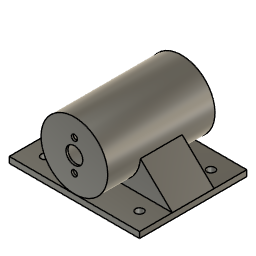
motor_support_v6 (Autodesk Fusion 360 design; units mm, degrees)
Autodesk Fusion 360 part; units mm, degrees
note: some values were not read from the file. Set by a fixed rule: which sketch regions a step uses.
sketch "Esboço1" plane through (0, 0, 0) normal (0, 1, 0) x (1, 0, 0)
  circle A0 centre (0, 7.75) radius 1.5
  circle A1 centre (0, -7.75) radius 1.5
  circle A2 centre (0, -0.0264) radius 4.25
  line L0 (0, 9.25) -> (0, 13.2236) construction
  line L1 (4.2485, 0.0836) -> (13.2495, 0.0836) construction
  line L2 (-4.2485, 0.0836) -> (-13.2495, 0.0836) construction
  line L3 (0.0108, -13.2764) -> (0.0108, -9.25) construction
  line L4 (0.0108, -6.25) -> (0.0108, -4.2764) construction
  line L5 (0.0108, 6.25) -> (0.0108, 4.2235) construction
  circle A3 centre (0, -0.0264) radius 14.25
  dimension "d3" = 3
  dimension "d5" = 3
  dimension "d73" = 8.4999
  dimension "d79" = 9.001
  dimension "d80" = 9.001
  dimension "d81" = 4.0265
  dimension "d82" = 1.9737
  dimension "d83" = 2.0265
  dimension "d84" = 3.9736
  dimension "d269" = 28.5
  constraint coincident A0 L0.start
  constraint vertical L0
  constraint coincident A2 L1.start
  constraint horizontal L1
  constraint coincident A2 L2.start
  constraint parallel L1 L2
  constraint coincident A1 L3.end
  constraint vertical L3
  constraint coincident A1 L4.start
  constraint coincident A2 L4.end
  constraint parallel L3 L4
  constraint coincident A0 L5.start
  constraint coincident A2 L5.end
  constraint parallel L4 L5
  measures "d3" diameter of A0
  measures "d5" diameter of A1
  measures "d73" diameter of A2
  measures "d79" distance of L1.start L1.end
  measures "d80" distance of L2.start L2.end
  measures "d81" distance of L3.start L3.end
  measures "d82" distance of L4.start L4.end
  measures "d83" distance of L5.start L5.end
  measures "d84" distance of L0.start L0.end
  measures "d269" diameter of A3
sketch "Esboço8" plane through (0, 0, 0) normal (0, 1, 0) x (1, 0, 0)
  circle A0 centre (0, 0) radius 16.8
  dimension "d87" = 33.6
  constraint coincident A0.centre origin
  measures "d87" diameter of A0
extrude "Extrusão14" add sketch "Esboço1" along normal blind 1
extrude "Extrusão15" add sketch "Esboço8" along normal blind 54 thin wall 3 inside
ref_plane "Plano de trabalho5" through (0, 27, 0) normal (0, 1, 0) x (1, 0, 0)
ref_plane "Plano de trabalho7" through (0, 33.6131, -16.8) normal (0, 0, -1) x (1, 0, 0)
sketch "Esboço14" plane through (0, 0, -16.8) normal (0, 0, -1) x (-1, 0, 0)
  line L0 (0, 0) -> (-15.8, 0)
  line L1 (0, 0) -> (15.8, 0)
  line L2 (0, 54) -> (-15.8, 54)
  line L3 (0, 54) -> (15.8, 54)
  line L4 (-15.8, 0) -> (-15.8, 54) construction
  line L5 (15.8, 0) -> (15.8, 54) construction
  line L6 (-15.8, 0) -> (-32.8, 0)
  line L7 (15.8, 0) -> (32.8, 0)
  line L8 (-15.8, 54) -> (-32.8, 54)
  line L9 (15.8, 54) -> (32.8, 54)
  line L10 (32.8, 0) -> (32.8, 54)
  line L11 (-32.8, 0) -> (-32.8, 54)
  line L12 (-32.8, 3) -> (-29.8, 3) construction
  line L13 (-29.8, 0) -> (-29.8, 3) construction
  circle A0 centre (-23.8, 9) radius 6 construction
  circle A1 centre (-23.8, 9) radius 2
  line L14 (-32.8, 27) -> (32.8, 27) construction
  line L15 (-32.8, 27) -> (32.8, 27) construction
  circle A2 centre (-23.8, 45) radius 6 construction
  circle A3 centre (-23.8, 45) radius 2
  line L16 (-29.8, 54) -> (-29.8, 51) construction
  line L17 (-32.8, 51) -> (-29.8, 51) construction
  line L18 (0, 0) -> (0, 54) construction
  circle A4 centre (23.8, 9) radius 2
  circle A5 centre (23.8, 9) radius 6 construction
  line L19 (32.8, 3) -> (29.8, 3) construction
  line L20 (29.8, 0) -> (29.8, 3) construction
  circle A6 centre (23.8, 45) radius 6 construction
  circle A7 centre (23.8, 45) radius 2
  line L21 (32.8, 51) -> (29.8, 51) construction
  line L22 (29.8, 54) -> (29.8, 51) construction
  dimension "d244" = 15.8
  dimension "d245" = 15.8
  dimension "d246" = 15.8
  dimension "d247" = 15.8
  dimension "d249" = 17
  dimension "d250" = 17
  dimension "d251" = 17
  dimension "d252" = 17
  dimension "d253" = 54
  dimension "d256" = 6
  dimension "d257" = 4
  dimension "d258" = 3
  dimension "d259" = 3
  constraint coincident L0.start L1.start
  constraint horizontal L0
  constraint parallel L0 L1
  constraint horizontal L2
  constraint parallel L2 L3
  constraint perpendicular L2 L4
  constraint perpendicular L4 L6
  constraint perpendicular L5 L7
  constraint perpendicular L4 L8
  constraint perpendicular L5 L9
  constraint coincident L11 L12.start
  constraint coincident L6 L13.start
  constraint perpendicular L12 L13
  constraint tangent L13 A0
  constraint concentric A0 A1
  constraint midpoint L11 L14.start
  constraint midpoint L10 L14.end
  constraint symmetric L12.start L14 L17.start
  constraint symmetric L12.end L14 L16.end
  constraint symmetric L13.start L14 L16.start
  constraint symmetric A0 L14 A2
  constraint symmetric A1 L14 A3
  constraint symmetric L15.start L14 L14.start
  constraint symmetric L15.end L14 L14.end
  constraint symmetric L12.start L18 L19.start
  constraint symmetric L12.end L18 L19.end
  constraint symmetric L13.start L18 L20.start
  constraint symmetric A0 L18 A5
  constraint symmetric A1 L18 A4
  constraint symmetric A2 L18 A6
  constraint symmetric A3 L18 A7
  constraint symmetric L16.start L18 L22.start
  constraint symmetric L16.end L18 L21.end
  constraint symmetric L17.start L18 L21.start
  measures "d244" distance of L0.start L0.end
  measures "d245" distance of L0.start L1.end
  measures "d246" distance of L2.start L2.end
  measures "d247" distance of L2.start L3.end
  measures "d249" distance of L0.end L6.end
  measures "d250" distance of L1.end L7.end
  measures "d251" distance of L2.end L8.end
  measures "d252" distance of L3.end L9.end
  measures "d253" distance of L6.end L8.end
  measures "d256" radius of A0
  measures "d257" diameter of A1
  measures "d258" distance of L12.end L13.start
  measures "d259" distance of L12.start L12.end
extrude "Extrusão19" add sketch "Esboço14" along normal blind 3
sketch "Esboço16" plane through (0, 27, 0) normal (0, 1, 0) x (1, 0, 0)
  line L0 (-15.7624, 0.308) -> (-15.7658, 1.0442) construction
  line L1 (-15.7658, 1.0442) -> (-15.5807, 1.9927) construction
  line L2 (-15.5807, 1.9927) -> (-15.3833, 3.1059) construction
  line L3 (-15.3833, 3.1059) -> (-14.9922, 4.8134) construction
  line L4 (-14.9922, 4.8134) -> (-14.4953, 6.3301) construction
  line L5 (-14.4953, 6.3301) -> (-13.9136, 7.4073) construction
  line L6 (-13.9136, 7.4073) -> (-13.3147, 8.5185) construction
  spline S0 degree 5 poles (-15.7624, 0.308) (-15.7658, 1.0442) (-15.5807, 1.9927) (-15.3833, 3.1059) (-14.9922, 4.8134) (-14.4953, 6.3301) (-13.9136, 7.4073) (-13.3147, 8.5185) knots 0 0 0 0 0 0 0.333333 0.666667 1 1 1 1 1 1
  line L7 (-13.3147, 8.5185) -> (-12.808, 9.3377) construction
  line L8 (-12.808, 9.3377) -> (-12.1195, 10.2348) construction
  line L9 (-12.1195, 10.2348) -> (-11.5134, 10.9511) construction
  line L10 (-11.5134, 10.9511) -> (-11.1095, 11.3586) construction
  line L11 (-11.1095, 11.3586) -> (-10.419, 11.9608) construction
  line L12 (-10.419, 11.9608) -> (-9.5369, 12.6651) construction
  line L13 (-9.5369, 12.6651) -> (-8.6927, 13.3173) construction
  line L14 (-8.6927, 13.3173) -> (-7.1711, 14.2921) construction
  line L15 (-7.1711, 14.2921) -> (-6.2997, 14.7005) construction
  line L16 (-6.2997, 14.7005) -> (-5.1953, 15.1411) construction
  line L17 (-5.1953, 15.1411) -> (-4.2429, 15.463) construction
  line L18 (-4.2429, 15.463) -> (-2.9702, 15.8824) construction
  line L19 (-2.9702, 15.8824) -> (-1.4208, 16.2541) construction
  line L20 (-1.4208, 16.2541) -> (-1.8542, 16.2524) construction
  line L21 (-1.8542, 16.2524) -> (0.5507, 16.8024) construction
  spline S1 degree 5 poles (-13.3147, 8.5185) (-12.808, 9.3377) (-12.1195, 10.2348) (-11.5134, 10.9511) (-11.1095, 11.3586) (-10.419, 11.9608) (-9.5369, 12.6651) (-8.6927, 13.3173) (-7.1711, 14.2921) (-6.2997, 14.7005) (-5.1953, 15.1411) (-4.2429, 15.463) (-2.9702, 15.8824) (-1.4208, 16.2541) (-1.8542, 16.2524) (0.5507, 16.8024) knots 0 0 0 0 0 0 0.090909 0.181818 0.272727 0.363636 0.454545 0.545455 0.636364 0.727273 0.818182 0.909091 1 1 1 1 1 1
  line L22 (0.5507, 16.8024) -> (-32.8128, 16.8024)
  line L23 (-32.8128, 16.8024) -> (-15.7624, 0.308)
  line L24 (0, 0) -> (0, 35) construction
  line L25 (-0.5507, 16.8024) -> (32.8128, 16.8024)
  line L26 (32.8128, 16.8024) -> (15.7624, 0.308)
  line L27 (15.7624, 0.308) -> (15.7677, 1.0369) construction
  line L28 (15.7677, 1.0369) -> (15.6756, 2.0308) construction
  line L29 (15.6756, 2.0308) -> (15.489, 2.9979) construction
  line L30 (15.489, 2.9979) -> (15.2883, 4.0369) construction
  line L31 (15.2883, 4.0369) -> (14.8066, 5.5314) construction
  line L32 (14.8066, 5.5314) -> (14.2143, 6.9545) construction
  line L33 (14.2143, 6.9545) -> (13.834, 7.6293) construction
  line L34 (13.834, 7.6293) -> (13.2272, 8.6663) construction
  line L35 (13.2272, 8.6663) -> (12.7561, 9.3389) construction
  line L36 (12.7561, 9.3389) -> (12.2228, 10.105) construction
  line L37 (12.2228, 10.105) -> (11.5429, 10.9084) construction
  line L38 (11.5429, 10.9084) -> (10.2941, 12.2432) construction
  line L39 (10.2941, 12.2432) -> (9.2906, 13.0216) construction
  line L40 (9.2906, 13.0216) -> (7.5196, 14.3421) construction
  line L41 (7.5196, 14.3421) -> (6.5603, 14.8819) construction
  line L42 (6.5603, 14.8819) -> (4.9642, 15.708) construction
  line L43 (4.9642, 15.708) -> (2.9932, 16.5653) construction
  line L44 (2.9932, 16.5653) -> (1.7822, 16.8024) construction
  line L45 (1.7822, 16.8024) -> (0.5507, 16.8024) construction
  line L46 (0.5507, 16.8024) -> (0.3206, 16.8024) construction
  spline S2 degree 5 poles (15.7624, 0.308) (15.7677, 1.0369) (15.6756, 2.0308) (15.489, 2.9979) (15.2883, 4.0369) (14.8066, 5.5314) (14.2143, 6.9545) (13.834, 7.6293) (13.2272, 8.6663) (12.7561, 9.3389) (12.2228, 10.105) (11.5429, 10.9084) (10.2941, 12.2432) (9.2906, 13.0216) (7.5196, 14.3421) (6.5603, 14.8819) (4.9642, 15.708) (2.9932, 16.5653) (1.7822, 16.8024) (0.5507, 16.8024) (0.3206, 16.8024) knots 0 0 0 0 0 0 0.0625 0.125 0.1875 0.25 0.3125 0.375 0.4375 0.5 0.5625 0.625 0.6875 0.75 0.8125 0.875 0.9375 1 1 1 1 1 1
  constraint coincident L24.start origin
  constraint perpendicular L22 L24
  constraint symmetric L22.end L24 L25.end
  constraint symmetric L0.start L24 L26.end
  constraint symmetric L21.end L24 L25.start
  constraint coincident L21.end S1.end
  constraint coincident L46.end L45
  constraint coincident L25 L44.end
extrude "Extrusão20" add sketch "Esboço16" along normal mid plane 21 contours L25 L26 S2
extrude "Extrusão21" add sketch "Esboço16" along normal mid plane 21 contours S0 S1 L22 L23 L25 S2
